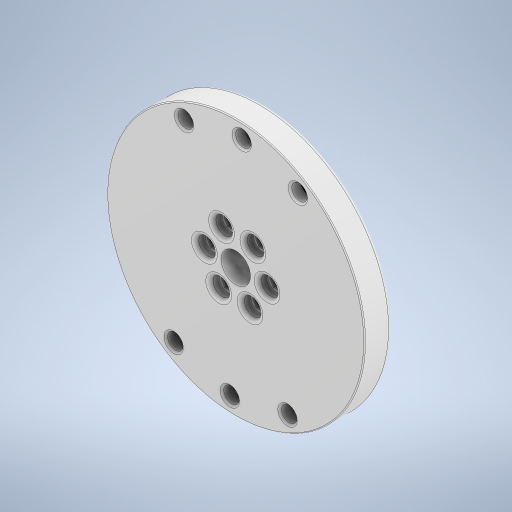
# Autodesk Inventor part: Góra
Saved by Autodesk Inventor 2023 (Build 270158000, 158)
## iProperties
Created: 2022-12-12
Part Number: Góra
Material: Stal, stopowa
Document SubType Name: Modeling
Designer: komputer
Density: 7.73 g/cm^3
Appearance: Gładki — biały
Author: komputer
Autodesk Inventor part; units mm, degrees
(part 1 of 2)
ref_plane "YZ Plane" through (0, 0, 0) normal (1, 0, 0) x (0, 1, 0)
ref_plane "XZ Plane" through (0, 0, 0) normal (0, 1, 0) x (-1, 0, 0)
sketch "Sketch1" plane through (0, 0, 0) normal (0, 0, 1) x (1, 0, 0)
  circle A0 centre (-9.064195, 40.309091) radius 2
  circle A1 centre (-10.61138, 10.787058) radius 2
  circle A2 centre (15.729043, 24.208174) radius 2
  circle A3 centre (6.433174, 9.893791) radius 2
  circle A4 centre (-18.360064, 25.994708) radius 2
  circle A5 centre (7.980358, 39.415824) radius 2
  circle A6 centre (-1.315511, 25.101441) radius 9
  circle A7 centre (-1.315511, 25.101441) radius 24.135889
  circle A8 centre (-1.315511, 25.101441) radius 25
  circle A9 centre (-9.064195, 40.309091) radius 3.5
  circle A10 centre (-10.61138, 10.787058) radius 3.5
  circle A11 centre (15.729043, 24.208174) radius 3.5
  circle A12 centre (6.433174, 9.893791) radius 3.5
  circle A13 centre (-18.360064, 25.994708) radius 3.5
  circle A14 centre (7.980358, 39.415824) radius 3.5
  arc A15 (-0.870133, 59.093921) -> (-1.760889, 59.093921) centre (-1.315511, 25.101441) ccw
  arc A16 (1.794733, 58.954262) -> (-0.870133, 59.093921) centre (-1.315511, 25.101441) ccw
  arc A17 (2.680609, 58.861152) -> (1.794733, 58.954262) centre (-1.315511, 25.101441) ccw
  arc A18 (5.316278, 58.443703) -> (2.680609, 58.861152) centre (-1.315511, 25.101441) ccw
  arc A19 (6.187569, 58.258505) -> (5.316278, 58.443703) centre (-1.315511, 25.101441) ccw
  arc A20 (8.765164, 57.56784) -> (6.187569, 58.258505) centre (-1.315511, 25.101441) ccw
  arc A21 (9.612323, 57.292581) -> (8.765164, 57.56784) centre (-1.315511, 25.101441) ccw
  arc A22 (12.103603, 56.336269) -> (9.612323, 57.292581) centre (-1.315511, 25.101441) ccw
  arc A23 (12.91735, 55.973965) -> (12.103603, 56.336269) centre (-1.315511, 25.101441) ccw
  arc A24 (15.295021, 54.762481) -> (12.91735, 55.973965) centre (-1.315511, 25.101441) ccw
  arc A25 (16.066438, 54.317103) -> (15.295021, 54.762481) centre (-1.315511, 25.101441) ccw
  arc A26 (18.304449, 52.863722) -> (16.066438, 54.317103) centre (-1.315511, 25.101441) ccw
  arc A27 (19.025086, 52.340149) -> (18.304449, 52.863722) centre (-1.315511, 25.101441) ccw
  arc A28 (21.098918, 50.660793) -> (19.025086, 52.340149) centre (-1.315511, 25.101441) ccw
  arc A29 (21.760878, 50.064761) -> (21.098918, 50.660793) centre (-1.315511, 25.101441) ccw
  arc A30 (23.647809, 48.17783) -> (21.760878, 50.064761) centre (-1.315511, 25.101441) ccw
  arc A31 (24.243841, 47.51587) -> (23.647809, 48.17783) centre (-1.315511, 25.101441) ccw
  arc A32 (25.923197, 45.442038) -> (24.243841, 47.51587) centre (-1.315511, 25.101441) ccw
  arc A33 (26.44677, 44.721401) -> (25.923197, 45.442038) centre (-1.315511, 25.101441) ccw
  arc A34 (27.900152, 42.48339) -> (26.44677, 44.721401) centre (-1.315511, 25.101441) ccw
  arc A35 (28.34553, 41.711972) -> (27.900152, 42.48339) centre (-1.315511, 25.101441) ccw
  arc A36 (29.557014, 39.334301) -> (28.34553, 41.711972) centre (-1.315511, 25.101441) ccw
  arc A37 (29.919317, 38.520555) -> (29.557014, 39.334301) centre (-1.315511, 25.101441) ccw
  arc A38 (30.87563, 36.029275) -> (29.919317, 38.520555) centre (-1.315511, 25.101441) ccw
  arc A39 (31.150888, 35.182115) -> (30.87563, 36.029275) centre (-1.315511, 25.101441) ccw
  arc A40 (31.841553, 32.604521) -> (31.150888, 35.182115) centre (-1.315511, 25.101441) ccw
  arc A41 (32.026751, 31.73323) -> (31.841553, 32.604521) centre (-1.315511, 25.101441) ccw
  arc A42 (32.4442, 29.097561) -> (32.026751, 31.73323) centre (-1.315511, 25.101441) ccw
  arc A43 (32.53731, 28.211685) -> (32.4442, 29.097561) centre (-1.315511, 25.101441) ccw
  arc A44 (32.676969, 25.546819) -> (32.53731, 28.211685) centre (-1.315511, 25.101441) ccw
  arc A45 (32.676969, 24.656063) -> (32.676969, 25.546819) centre (-1.315511, 25.101441) ccw
  arc A46 (32.53731, 21.991198) -> (32.676969, 24.656063) centre (-1.315511, 25.101441) ccw
  arc A47 (32.4442, 21.105321) -> (32.53731, 21.991198) centre (-1.315511, 25.101441) ccw
  arc A48 (32.026751, 18.469653) -> (32.4442, 21.105321) centre (-1.315511, 25.101441) ccw
  arc A49 (31.841553, 17.598362) -> (32.026751, 18.469653) centre (-1.315511, 25.101441) ccw
  arc A50 (31.150888, 15.020767) -> (31.841553, 17.598362) centre (-1.315511, 25.101441) ccw
  arc A51 (30.87563, 14.173607) -> (31.150888, 15.020767) centre (-1.315511, 25.101441) ccw
  arc A52 (29.919317, 11.682327) -> (30.87563, 14.173607) centre (-1.315511, 25.101441) ccw
  arc A53 (29.557014, 10.868581) -> (29.919317, 11.682327) centre (-1.315511, 25.101441) ccw
  arc A54 (28.34553, 8.49091) -> (29.557014, 10.868581) centre (-1.315511, 25.101441) ccw
  arc A55 (27.900152, 7.719492) -> (28.34553, 8.49091) centre (-1.315511, 25.101441) ccw
  arc A56 (26.44677, 5.481481) -> (27.900152, 7.719492) centre (-1.315511, 25.101441) ccw
  arc A57 (25.923197, 4.760844) -> (26.44677, 5.481481) centre (-1.315511, 25.101441) ccw
  arc A58 (24.243841, 2.687013) -> (25.923197, 4.760844) centre (-1.315511, 25.101441) ccw
  arc A59 (23.647809, 2.025052) -> (24.243841, 2.687013) centre (-1.315511, 25.101441) ccw
  arc A60 (21.760878, 0.138121) -> (23.647809, 2.025052) centre (-1.315511, 25.101441) ccw
  arc A61 (21.098918, -0.457911) -> (21.760878, 0.138121) centre (-1.315511, 25.101441) ccw
  arc A62 (19.025086, -2.137266) -> (21.098918, -0.457911) centre (-1.315511, 25.101441) ccw
  arc A63 (18.304449, -2.66084) -> (19.025086, -2.137266) centre (-1.315511, 25.101441) ccw
  arc A64 (16.066438, -4.114221) -> (18.304449, -2.66084) centre (-1.315511, 25.101441) ccw
  arc A65 (15.295021, -4.559599) -> (16.066438, -4.114221) centre (-1.315511, 25.101441) ccw
  arc A66 (12.91735, -5.771083) -> (15.295021, -4.559599) centre (-1.315511, 25.101441) ccw
  arc A67 (12.103603, -6.133386) -> (12.91735, -5.771083) centre (-1.315511, 25.101441) ccw
  arc A68 (9.612323, -7.089699) -> (12.103603, -6.133386) centre (-1.315511, 25.101441) ccw
  arc A69 (8.765164, -7.364958) -> (9.612323, -7.089699) centre (-1.315511, 25.101441) ccw
  arc A70 (6.187569, -8.055623) -> (8.765164, -7.364958) centre (-1.315511, 25.101441) ccw
  arc A71 (5.316278, -8.240821) -> (6.187569, -8.055623) centre (-1.315511, 25.101441) ccw
  arc A72 (2.680609, -8.65827) -> (5.316278, -8.240821) centre (-1.315511, 25.101441) ccw
  arc A73 (1.794733, -8.751379) -> (2.680609, -8.65827) centre (-1.315511, 25.101441) ccw
  arc A74 (-0.870133, -8.891039) -> (1.794733, -8.751379) centre (-1.315511, 25.101441) ccw
  arc A75 (-1.760889, -8.891039) -> (-0.870133, -8.891039) centre (-1.315511, 25.101441) ccw
  arc A76 (-4.425754, -8.751379) -> (-1.760889, -8.891039) centre (-1.315511, 25.101441) ccw
  arc A77 (-5.311631, -8.65827) -> (-4.425754, -8.751379) centre (-1.315511, 25.101441) ccw
  arc A78 (-7.947299, -8.240821) -> (-5.311631, -8.65827) centre (-1.315511, 25.101441) ccw
  arc A79 (-8.81859, -8.055623) -> (-7.947299, -8.240821) centre (-1.315511, 25.101441) ccw
  arc A80 (-11.396185, -7.364958) -> (-8.81859, -8.055623) centre (-1.315511, 25.101441) ccw
  arc A81 (-12.243345, -7.089699) -> (-11.396185, -7.364958) centre (-1.315511, 25.101441) ccw
  arc A82 (-14.734625, -6.133386) -> (-12.243345, -7.089699) centre (-1.315511, 25.101441) ccw
  arc A83 (-15.548371, -5.771083) -> (-14.734625, -6.133386) centre (-1.315511, 25.101441) ccw
  arc A84 (-17.926042, -4.559599) -> (-15.548371, -5.771083) centre (-1.315511, 25.101441) ccw
  arc A85 (-18.69746, -4.114221) -> (-17.926042, -4.559599) centre (-1.315511, 25.101441) ccw
  arc A86 (-20.935471, -2.66084) -> (-18.69746, -4.114221) centre (-1.315511, 25.101441) ccw
  arc A87 (-21.656108, -2.137266) -> (-20.935471, -2.66084) centre (-1.315511, 25.101441) ccw
  arc A88 (-23.729939, -0.457911) -> (-21.656108, -2.137266) centre (-1.315511, 25.101441) ccw
  arc A89 (-24.3919, 0.138121) -> (-23.729939, -0.457911) centre (-1.315511, 25.101441) ccw
  arc A90 (-26.27883, 2.025052) -> (-24.3919, 0.138121) centre (-1.315511, 25.101441) ccw
  arc A91 (-26.874863, 2.687013) -> (-26.27883, 2.025052) centre (-1.315511, 25.101441) ccw
  arc A92 (-28.554218, 4.760844) -> (-26.874863, 2.687013) centre (-1.315511, 25.101441) ccw
  arc A93 (-29.077792, 5.481481) -> (-28.554218, 4.760844) centre (-1.315511, 25.101441) ccw
  arc A94 (-30.531173, 7.719492) -> (-29.077792, 5.481481) centre (-1.315511, 25.101441) ccw
  arc A95 (-30.976551, 8.49091) -> (-30.531173, 7.719492) centre (-1.315511, 25.101441) ccw
  arc A96 (-32.188035, 10.868581) -> (-30.976551, 8.49091) centre (-1.315511, 25.101441) ccw
  arc A97 (-32.550338, 11.682327) -> (-32.188035, 10.868581) centre (-1.315511, 25.101441) ccw
  arc A98 (-33.506651, 14.173607) -> (-32.550338, 11.682327) centre (-1.315511, 25.101441) ccw
  arc A99 (-33.78191, 15.020767) -> (-33.506651, 14.173607) centre (-1.315511, 25.101441) ccw
  arc A100 (-34.472574, 17.598362) -> (-33.78191, 15.020767) centre (-1.315511, 25.101441) ccw
  arc A101 (-34.657773, 18.469653) -> (-34.472574, 17.598362) centre (-1.315511, 25.101441) ccw
  arc A102 (-35.075222, 21.105321) -> (-34.657773, 18.469653) centre (-1.315511, 25.101441) ccw
  arc A103 (-35.168331, 21.991198) -> (-35.075222, 21.105321) centre (-1.315511, 25.101441) ccw
  arc A104 (-35.307991, 24.656063) -> (-35.168331, 21.991198) centre (-1.315511, 25.101441) ccw
  arc A105 (-35.307991, 25.546819) -> (-35.307991, 24.656063) centre (-1.315511, 25.101441) ccw
  arc A106 (-35.168331, 28.211685) -> (-35.307991, 25.546819) centre (-1.315511, 25.101441) ccw
  arc A107 (-35.075222, 29.097561) -> (-35.168331, 28.211685) centre (-1.315511, 25.101441) ccw
  arc A108 (-34.657773, 31.73323) -> (-35.075222, 29.097561) centre (-1.315511, 25.101441) ccw
  arc A109 (-34.472574, 32.604521) -> (-34.657773, 31.73323) centre (-1.315511, 25.101441) ccw
  arc A110 (-33.78191, 35.182115) -> (-34.472574, 32.604521) centre (-1.315511, 25.101441) ccw
  arc A111 (-33.506651, 36.029275) -> (-33.78191, 35.182115) centre (-1.315511, 25.101441) ccw
  arc A112 (-32.550338, 38.520555) -> (-33.506651, 36.029275) centre (-1.315511, 25.101441) ccw
  arc A113 (-32.188035, 39.334301) -> (-32.550338, 38.520555) centre (-1.315511, 25.101441) ccw
  arc A114 (-30.976551, 41.711972) -> (-32.188035, 39.334301) centre (-1.315511, 25.101441) ccw
  arc A115 (-30.531173, 42.48339) -> (-30.976551, 41.711972) centre (-1.315511, 25.101441) ccw
  arc A116 (-29.077792, 44.721401) -> (-30.531173, 42.48339) centre (-1.315511, 25.101441) ccw
  arc A117 (-28.554218, 45.442038) -> (-29.077792, 44.721401) centre (-1.315511, 25.101441) ccw
  arc A118 (-26.874863, 47.51587) -> (-28.554218, 45.442038) centre (-1.315511, 25.101441) ccw
  arc A119 (-26.27883, 48.17783) -> (-26.874863, 47.51587) centre (-1.315511, 25.101441) ccw
  arc A120 (-24.3919, 50.064761) -> (-26.27883, 48.17783) centre (-1.315511, 25.101441) ccw
  arc A121 (-23.729939, 50.660793) -> (-24.3919, 50.064761) centre (-1.315511, 25.101441) ccw
  arc A122 (-21.656108, 52.340149) -> (-23.729939, 50.660793) centre (-1.315511, 25.101441) ccw
  arc A123 (-20.935471, 52.863722) -> (-21.656108, 52.340149) centre (-1.315511, 25.101441) ccw
  arc A124 (-18.69746, 54.317103) -> (-20.935471, 52.863722) centre (-1.315511, 25.101441) ccw
  arc A125 (-17.926042, 54.762481) -> (-18.69746, 54.317103) centre (-1.315511, 25.101441) ccw
  arc A126 (-15.548371, 55.973965) -> (-17.926042, 54.762481) centre (-1.315511, 25.101441) ccw
  arc A127 (-14.734625, 56.336269) -> (-15.548371, 55.973965) centre (-1.315511, 25.101441) ccw
  arc A128 (-12.243345, 57.292581) -> (-14.734625, 56.336269) centre (-1.315511, 25.101441) ccw
  arc A129 (-11.396185, 57.56784) -> (-12.243345, 57.292581) centre (-1.315511, 25.101441) ccw
  arc A130 (-8.81859, 58.258505) -> (-11.396185, 57.56784) centre (-1.315511, 25.101441) ccw
  arc A131 (-7.947299, 58.443703) -> (-8.81859, 58.258505) centre (-1.315511, 25.101441) ccw
  arc A132 (-5.311631, 58.861152) -> (-7.947299, 58.443703) centre (-1.315511, 25.101441) ccw
  arc A133 (-4.425754, 58.954262) -> (-5.311631, 58.861152) centre (-1.315511, 25.101441) ccw
  arc A134 (-1.760889, 59.093921) -> (-4.425754, 58.954262) centre (-1.315511, 25.101441) ccw
  circle A135 centre (-1.315511, 25.101441) radius 9
  circle A136 centre (-1.315511, 25.101441) radius 8
  point P0 (0, 0)
extrude "Extrusion1" add sketch "Sketch1" along normal blind 37 contours A6 | A7 | A9 | A10 | A11 | A12 | A13 | A14
sketch "Sketch2" plane through (-1.315511, 25.101441, 37) normal (0, 0, 1) x (1, 0, 0)
  circle A0 centre (0, 0) radius 43.680391
  circle A1 centre (0, 0) radius 8
  circle A2 centre (0, 0) radius 50
  circle A3 centre (0, 0) radius 24.135889
  circle A4 centre (9.295869, 14.314383) radius 2
  circle A5 centre (-17.044553, 0.893267) radius 2
  circle A6 centre (7.748685, -15.20765) radius 2
  circle A7 centre (17.044553, -0.893267) radius 2
  circle A8 centre (-9.295869, -14.314383) radius 2
  circle A9 centre (-7.748685, 15.20765) radius 2
  circle A10 centre (0, 0) radius 8
  point P0 (1.315511, -25.101441)
  dimension "d2" = 100
  constraints: 1 centre point, 1 coincident
  measures "d2" diameter of A2
extrude "Extrusion2" add sketch "Sketch2" against normal blind 10 contours A0 | A2
sketch "Sketch3" plane through (-1.315511, 25.101441, 37) normal (0, 0, 1) x (1, 0, 0)
  circle A0 centre (0, 0) radius 55
  circle A1 centre (0, 0) radius 50
  circle A2 centre (9.295869, 14.314383) radius 2
  circle A3 centre (-17.044553, 0.893267) radius 2
  circle A4 centre (7.748685, -15.20765) radius 2
  circle A5 centre (17.044553, -0.893267) radius 2
  circle A6 centre (-9.295869, -14.314383) radius 2
  circle A7 centre (-7.748685, 15.20765) radius 2
  circle A8 centre (0, 0) radius 8
  point P0 (1.315511, -25.101441)
  constraints: 1 centre point, 2 other
ref_plane "Work Plane1" through (-65.256929, -38.839977, 26) normal (0, 0, 1) x (0.9839108, 0.1786605, 0)
extrude "Extrusion3" add sketch "Sketch3" against normal blind 10 contours A0
sketch "Sketch4" plane through (-1.315511, 25.101441, 37) normal (0, 0, 1) x (1, 0, 0)
  circle A0 centre (0, 0) radius 55
  circle A1 centre (9.295869, 14.314383) radius 2
  circle A2 centre (-17.044553, 0.893267) radius 2
  circle A3 centre (7.748685, -15.20765) radius 2
  circle A4 centre (17.044553, -0.893267) radius 2
  circle A5 centre (-9.295869, -14.314383) radius 2
  circle A6 centre (-7.748685, 15.20765) radius 2
  circle A7 centre (0, 0) radius 8
  line L0 (-9.295869, -14.314383) -> (-9.295869, -10.814383)
  line L1 (-9.295869, -10.814383) -> (-9.295869, -17.414383)
  line L2 (-11.085655, -17.414383) -> (-12.87544, -14.314383)
  line L3 (-12.87544, -14.314383) -> (-11.085655, -11.214383)
  line L4 (-11.085655, -11.214383) -> (-7.506083, -11.214383)
  line L5 (-7.506083, -11.214383) -> (-5.716297, -14.314383)
  line L6 (-5.716297, -14.314383) -> (-7.506083, -17.414383)
  line L7 (-7.506083, -17.414383) -> (-11.085655, -17.414383)
  line L8 (9.53847, -12.10765) -> (11.328256, -15.20765)
  line L9 (9.53847, -18.30765) -> (5.958899, -18.30765)
  line L10 (5.958899, -18.30765) -> (4.169113, -15.20765)
  line L11 (11.328256, -15.20765) -> (9.53847, -18.30765)
  line L12 (4.169113, -15.20765) -> (5.958899, -12.10765)
  line L13 (5.958899, -12.10765) -> (9.53847, -12.10765)
  line L14 (15.254768, 2.206733) -> (18.834339, 2.206733)
  line L15 (20.624125, -0.893267) -> (18.834339, -3.993267)
  line L16 (18.834339, -3.993267) -> (15.254768, -3.993267)
  line L17 (18.834339, 2.206733) -> (20.624125, -0.893267)
  line L18 (15.254768, -3.993267) -> (13.464982, -0.893267)
  line L19 (13.464982, -0.893267) -> (15.254768, 2.206733)
  line L20 (5.716297, 14.314383) -> (7.506083, 17.414383)
  line L21 (11.085655, 17.414383) -> (12.87544, 14.314383)
  line L22 (12.87544, 14.314383) -> (11.085655, 11.214383)
  line L23 (7.506083, 17.414383) -> (11.085655, 17.414383)
  line L24 (11.085655, 11.214383) -> (7.506083, 11.214383)
  line L25 (7.506083, 11.214383) -> (5.716297, 14.314383)
  line L26 (-9.53847, 12.10765) -> (-11.328256, 15.20765)
  line L27 (-9.53847, 18.30765) -> (-5.958899, 18.30765)
  line L28 (-5.958899, 18.30765) -> (-4.169113, 15.20765)
  line L29 (-11.328256, 15.20765) -> (-9.53847, 18.30765)
  line L30 (-4.169113, 15.20765) -> (-5.958899, 12.10765)
  line L31 (-5.958899, 12.10765) -> (-9.53847, 12.10765)
  line L32 (-15.254768, -2.206733) -> (-18.834339, -2.206733)
  line L33 (-20.624125, 0.893267) -> (-18.834339, 3.993267)
  line L34 (-18.834339, 3.993267) -> (-15.254768, 3.993267)
  line L35 (-18.834339, -2.206733) -> (-20.624125, 0.893267)
  line L36 (-15.254768, 3.993267) -> (-13.464982, 0.893267)
  line L37 (-13.464982, 0.893267) -> (-15.254768, -2.206733)
  point P0 (1.315511, -25.101441)
  point P1 (10.433363, -16.75765)
  point P2 (7.748685, -15.20765)
  point P3 (4.717596, -13.45765)
  point P4 (19.729232, 0.656733)
  point P5 (17.044553, -0.893267)
  point P6 (14.013465, -2.643267)
  point P7 (9.295869, 17.414383)
  point P8 (9.295869, 14.314383)
  point P9 (9.295869, 10.814383)
  point P10 (-10.433363, 16.75765)
  point P11 (-7.748685, 15.20765)
  point P12 (-4.717596, 13.45765)
  point P13 (-19.729232, -0.656733)
  point P14 (-17.044553, 0.893267)
  point P15 (-14.013465, 2.643267)
  dimension "d7" = 3.5
  dimension "d8" = 6.6
  dimension "d11" = 360
  constraints: 76 end point, 2 coincident, 1 midpoint, 1 point on line, 1 vertical, 104 other
  measures "d7" distance of L0.start L0.end
  measures "d8" distance of L0.end L1.end
extrude "Extrusion4" cut sketch "Sketch4" against normal blind 5.4 contours A1 | A2 | A3 | A4 | A5 L1 L0 | A5 L0 L4 L5 L6 L7 L1 | L0 L1 A5 | A5 L1 L7 L2 L3 L4 L0 | A6 | L8 L11 L9 L10 L12 L13 | L14 L17 L15 L16 L18 L19 | L20 L23 L21 L22 L24 L25 | L26 L29 L27 L28 L30 L31 | L32 L35 L33 L34 L36 L37
sketch "Sketch14" plane through (-1.315511, 25.101441, 37) normal (0, 0, 1) x (1, 0, 0)
  circle A0 centre (0, 0) radius 55
  line L0 (-7.506083, -11.214383) -> (-5.716297, -14.314383)
  line L1 (-5.716297, -14.314383) -> (-7.506083, -17.414383)
  line L2 (-7.506083, -17.414383) -> (-11.085655, -17.414383)
  line L3 (-11.085655, -17.414383) -> (-12.87544, -14.314383)
  line L4 (-12.87544, -14.314383) -> (-11.085655, -11.214383)
  line L5 (-11.085655, -11.214383) -> (-7.506083, -11.214383)
  line L6 (18.834339, -3.993267) -> (15.254768, -3.993267)
  line L7 (15.254768, -3.993267) -> (13.464982, -0.893267)
  line L8 (13.464982, -0.893267) -> (15.254768, 2.206733)
  line L9 (15.254768, 2.206733) -> (18.834339, 2.206733)
  line L10 (18.834339, 2.206733) -> (20.624125, -0.893267)
  line L11 (20.624125, -0.893267) -> (18.834339, -3.993267)
  line L12 (12.87544, 14.314383) -> (11.085655, 11.214383)
  line L13 (11.085655, 11.214383) -> (7.506083, 11.214383)
  line L14 (7.506083, 11.214383) -> (5.716297, 14.314383)
  line L15 (5.716297, 14.314383) -> (7.506083, 17.414383)
  line L16 (7.506083, 17.414383) -> (11.085655, 17.414383)
  line L17 (11.085655, 17.414383) -> (12.87544, 14.314383)
  line L18 (-18.834339, 3.993267) -> (-15.254768, 3.993267)
  line L19 (-15.254768, 3.993267) -> (-13.464982, 0.893267)
  line L20 (-13.464982, 0.893267) -> (-15.254768, -2.206733)
  line L21 (-15.254768, -2.206733) -> (-18.834339, -2.206733)
  line L22 (-18.834339, -2.206733) -> (-20.624125, 0.893267)
  line L23 (-20.624125, 0.893267) -> (-18.834339, 3.993267)
  line L24 (5.958899, -18.30765) -> (4.169113, -15.20765)
  line L25 (4.169113, -15.20765) -> (5.958899, -12.10765)
  line L26 (5.958899, -12.10765) -> (9.53847, -12.10765)
  line L27 (9.53847, -12.10765) -> (11.328256, -15.20765)
  line L28 (11.328256, -15.20765) -> (9.53847, -18.30765)
  line L29 (9.53847, -18.30765) -> (5.958899, -18.30765)
  line L30 (-5.958899, 18.30765) -> (-4.169113, 15.20765)
  line L31 (-4.169113, 15.20765) -> (-5.958899, 12.10765)
  line L32 (-5.958899, 12.10765) -> (-9.53847, 12.10765)
  line L33 (-9.53847, 12.10765) -> (-11.328256, 15.20765)
  line L34 (-11.328256, 15.20765) -> (-9.53847, 18.30765)
  line L35 (-9.53847, 18.30765) -> (-5.958899, 18.30765)
  circle A1 centre (-9.295869, -14.314383) radius 2
  circle A2 centre (7.748685, -15.20765) radius 2
  circle A3 centre (9.295869, 14.314383) radius 2
  circle A4 centre (-7.748685, 15.20765) radius 2
  circle A5 centre (7.748685, -15.20765) radius 2
  line L36 (-9.295869, -14.314383) -> (7.748685, -15.20765)
  line L37 (-7.748685, 15.20765) -> (9.295869, 14.314383)
  line L38 (0, 0) -> (-0.773592, -14.761016)
  line L39 (0, 0) -> (0.773592, 14.761016)
  line L40 (0, 0) -> (2.355118, 44.938329)
  circle A6 centre (0, 0) radius 8
  line L41 (0, 0) -> (-2.355118, -44.938329)
  line L42 (-2.355118, -44.938329) -> (-54.509523, -42.205033)
  line L43 (-54.509523, -42.205033) -> (48.627627, -47.610222)
  line L44 (2.355118, 44.938329) -> (-54.509523, 47.918479)
  line L45 (2.355118, 44.938329) -> (72.939254, 41.239171)
  line L46 (2.355118, 44.938329) -> (3.506509, 66.908179)
  line L47 (0, 0) -> (-7.748685, 15.20765)
  line L48 (-7.748685, 15.20765) -> (-23.590038, 46.298057)
  line L49 (-23.590038, 46.298057) -> (-32.669848, 64.118188)
  circle A7 centre (0, 0) radius 71.961524
  circle A8 centre (-28.129943, 55.208122) radius 4
  circle A9 centre (-51.965307, 33.746665) radius 4
  circle A10 centre (-61.876608, 3.242816) radius 4
  circle A11 centre (-55.208122, -28.129943) radius 4
  circle A12 centre (-33.746665, -51.965307) radius 4
  circle A13 centre (-3.242816, -61.876608) radius 4
  circle A14 centre (28.129943, -55.208122) radius 4
  circle A15 centre (51.965307, -33.746665) radius 4
  circle A16 centre (61.876608, -3.242816) radius 4
  circle A17 centre (55.208122, 28.129943) radius 4
  circle A18 centre (33.746665, 51.965307) radius 4
  circle A19 centre (3.242816, 61.876608) radius 4
  line L50 (-2.355118, -44.938329) -> (-68.6558, -41.463658)
  line L51 (-68.6558, -41.463658) -> (71.961524, -48.833099)
  point P0 (1.315511, -25.101441)
  dimension "d60" = 45
  dimension "d61" = 45
  dimension "d62" = 22
  dimension "d63" = 20
  dimension "d65" = 8
  dimension "d69" = 360
  constraints: 32 end point, 12 centre point, 3 collinear, 3 midpoint, 3 perpendicular, 3 point on line, 2 coincident, 28 other
  measures "d60" distance of L38.start L40.end
  measures "d61" distance of L41.start L41.end
  measures "d62" distance of L40.end L46.end
  measures "d63" distance of L48.end L49.end
  measures "d65" diameter of A8
extrude "Extrusion16" add sketch "Sketch14" against normal up to surface (10 mm away) contours A0 L45 A7 L51 L43 | A0 L49 A8 A7 L45 | L43 L51 A7 L50 L42 A0 | L42 L50 A7 L44 A0 | A0 L44 A7 L49 A8 | A9 | A10 | A11 | A15 | A16 | A17
sketch "Sketch15" plane through (-1.315511, 25.101441, 37) normal (0, 0, 1) x (1, 0, 0)
  circle A0 centre (-28.129943, 55.208122) radius 4
  circle A1 centre (33.746665, 51.965307) radius 4
  circle A2 centre (-33.746665, -51.965307) radius 4
  circle A3 centre (-3.242816, -61.876608) radius 4
  circle A4 centre (28.129943, -55.208122) radius 4
  circle A5 centre (3.242816, 61.876608) radius 4
  circle A6 centre (0, 0) radius 71.961524
  line L0 (-7.506083, -11.214383) -> (-5.716297, -14.314383)
  line L1 (-5.716297, -14.314383) -> (-7.506083, -17.414383)
  line L2 (-7.506083, -17.414383) -> (-11.085655, -17.414383)
  line L3 (-11.085655, -17.414383) -> (-12.87544, -14.314383)
  line L4 (-12.87544, -14.314383) -> (-11.085655, -11.214383)
  line L5 (-11.085655, -11.214383) -> (-7.506083, -11.214383)
  line L6 (18.834339, -3.993267) -> (15.254768, -3.993267)
  line L7 (15.254768, -3.993267) -> (13.464982, -0.893267)
  line L8 (13.464982, -0.893267) -> (15.254768, 2.206733)
  line L9 (15.254768, 2.206733) -> (18.834339, 2.206733)
  line L10 (18.834339, 2.206733) -> (20.624125, -0.893267)
  line L11 (20.624125, -0.893267) -> (18.834339, -3.993267)
  line L12 (12.87544, 14.314383) -> (11.085655, 11.214383)
  line L13 (11.085655, 11.214383) -> (7.506083, 11.214383)
  line L14 (7.506083, 11.214383) -> (5.716297, 14.314383)
  line L15 (5.716297, 14.314383) -> (7.506083, 17.414383)
  line L16 (7.506083, 17.414383) -> (11.085655, 17.414383)
  line L17 (11.085655, 17.414383) -> (12.87544, 14.314383)
  line L18 (-18.834339, 3.993267) -> (-15.254768, 3.993267)
  line L19 (-15.254768, 3.993267) -> (-13.464982, 0.893267)
  line L20 (-13.464982, 0.893267) -> (-15.254768, -2.206733)
  line L21 (-15.254768, -2.206733) -> (-18.834339, -2.206733)
  line L22 (-18.834339, -2.206733) -> (-20.624125, 0.893267)
  line L23 (-20.624125, 0.893267) -> (-18.834339, 3.993267)
  line L24 (5.958899, -18.30765) -> (4.169113, -15.20765)
  line L25 (4.169113, -15.20765) -> (5.958899, -12.10765)
  line L26 (5.958899, -12.10765) -> (9.53847, -12.10765)
  line L27 (9.53847, -12.10765) -> (11.328256, -15.20765)
  line L28 (11.328256, -15.20765) -> (9.53847, -18.30765)
  line L29 (9.53847, -18.30765) -> (5.958899, -18.30765)
  line L30 (-5.958899, 18.30765) -> (-4.169113, 15.20765)
  line L31 (-4.169113, 15.20765) -> (-5.958899, 12.10765)
  line L32 (-5.958899, 12.10765) -> (-9.53847, 12.10765)
  line L33 (-9.53847, 12.10765) -> (-11.328256, 15.20765)
  line L34 (-11.328256, 15.20765) -> (-9.53847, 18.30765)
  line L35 (-9.53847, 18.30765) -> (-5.958899, 18.30765)
  circle A7 centre (0, 0) radius 70
  point P0 (1.315511, -25.101441)
  dimension "d73" = 140
  constraints: 1 centre point
  measures "d73" diameter of A7
extrude "Extrusion17" cut sketch "Sketch15" against normal through all contours A6
sketch "Sketch16" plane through (-1.315511, 25.101441, 27) normal (0, 0, -1) x (-1, 0, 0)
  circle A0 centre (0, 0) radius 70
  circle A1 centre (-3.242816, 61.876608) radius 4
  circle A2 centre (-28.129943, -55.208122) radius 4
  circle A3 centre (3.242816, -61.876608) radius 4
  circle A4 centre (33.746665, -51.965307) radius 4
  circle A5 centre (-33.746665, 51.965307) radius 4
  circle A6 centre (28.129943, 55.208122) radius 4
  circle A7 centre (0, 0) radius 24.135889
  circle A8 centre (-28.129943, -55.208122) radius 4
  circle A9 centre (28.129943, 55.208122) radius 4
  line L0 (-28.129943, -55.208122) -> (28.129943, 55.208122)
  line L1 (-28.129943, -55.208122) -> (-25.315202, -49.683882)
  line L2 (-22.125781, -51.308973) -> (-21.7511, -58.458305)
  line L3 (-21.7511, -58.458305) -> (-27.755263, -62.357454)
  line L4 (-27.755263, -62.357454) -> (-34.134106, -59.107271)
  line L5 (-34.134106, -59.107271) -> (-34.508787, -51.957939)
  line L6 (-34.508787, -51.957939) -> (-28.504624, -48.05879)
  line L7 (-28.504624, -48.05879) -> (-22.125781, -51.308973)
  line L8 (-0.656333, -55.872445) -> (6.492999, -55.497765)
  line L9 (-3.906516, -62.251289) -> (-0.656333, -55.872445)
  line L10 (-0.007367, -68.255452) -> (-3.906516, -62.251289)
  line L11 (7.141965, -67.880771) -> (-0.007367, -68.255452)
  line L12 (10.392148, -61.501927) -> (7.141965, -67.880771)
  line L13 (6.492999, -55.497765) -> (10.392148, -61.501927)
  line L14 (27.367821, -48.715124) -> (33.371984, -44.815975)
  line L15 (27.742502, -55.864456) -> (27.367821, -48.715124)
  line L16 (34.121345, -59.114639) -> (27.742502, -55.864456)
  line L17 (40.125508, -55.21549) -> (34.121345, -59.114639)
  line L18 (39.750828, -48.066158) -> (40.125508, -55.21549)
  line L19 (33.371984, -44.815975) -> (39.750828, -48.066158)
  line L20 (48.05879, -28.504624) -> (51.308973, -22.125781)
  line L21 (51.957939, -34.508787) -> (48.05879, -28.504624)
  line L22 (59.107271, -34.134106) -> (51.957939, -34.508787)
  line L23 (62.357454, -27.755263) -> (59.107271, -34.134106)
  line L24 (58.458305, -21.7511) -> (62.357454, -27.755263)
  line L25 (51.308973, -22.125781) -> (58.458305, -21.7511)
  line L26 (55.872445, -0.656333) -> (55.497765, 6.492999)
  line L27 (62.251289, -3.906516) -> (55.872445, -0.656333)
  line L28 (68.255452, -0.007367) -> (62.251289, -3.906516)
  line L29 (67.880771, 7.141965) -> (68.255452, -0.007367)
  line L30 (61.501927, 10.392148) -> (67.880771, 7.141965)
  line L31 (55.497765, 6.492999) -> (61.501927, 10.392148)
  line L32 (48.715124, 27.367821) -> (44.815975, 33.371984)
  line L33 (55.864456, 27.742502) -> (48.715124, 27.367821)
  line L34 (59.114639, 34.121345) -> (55.864456, 27.742502)
  line L35 (55.21549, 40.125508) -> (59.114639, 34.121345)
  line L36 (48.066158, 39.750828) -> (55.21549, 40.125508)
  line L37 (44.815975, 33.371984) -> (48.066158, 39.750828)
  line L38 (28.504624, 48.05879) -> (22.125781, 51.308973)
  line L39 (34.508787, 51.957939) -> (28.504624, 48.05879)
  line L40 (34.134106, 59.107271) -> (34.508787, 51.957939)
  line L41 (27.755263, 62.357454) -> (34.134106, 59.107271)
  line L42 (21.7511, 58.458305) -> (27.755263, 62.357454)
  line L43 (22.125781, 51.308973) -> (21.7511, 58.458305)
  line L44 (0.656333, 55.872445) -> (-6.492999, 55.497765)
  line L45 (3.906516, 62.251289) -> (0.656333, 55.872445)
  line L46 (0.007367, 68.255452) -> (3.906516, 62.251289)
  line L47 (-7.141965, 67.880771) -> (0.007367, 68.255452)
  line L48 (-10.392148, 61.501927) -> (-7.141965, 67.880771)
  line L49 (-6.492999, 55.497765) -> (-10.392148, 61.501927)
  line L50 (-27.367821, 48.715124) -> (-33.371984, 44.815975)
  line L51 (-27.742502, 55.864456) -> (-27.367821, 48.715124)
  line L52 (-34.121345, 59.114639) -> (-27.742502, 55.864456)
  line L53 (-40.125508, 55.21549) -> (-34.121345, 59.114639)
  line L54 (-39.750828, 48.066158) -> (-40.125508, 55.21549)
  line L55 (-33.371984, 44.815975) -> (-39.750828, 48.066158)
  line L56 (-48.05879, 28.504624) -> (-51.308973, 22.125781)
  line L57 (-51.957939, 34.508787) -> (-48.05879, 28.504624)
  line L58 (-59.107271, 34.134106) -> (-51.957939, 34.508787)
  line L59 (-62.357454, 27.755263) -> (-59.107271, 34.134106)
  line L60 (-58.458305, 21.7511) -> (-62.357454, 27.755263)
  line L61 (-51.308973, 22.125781) -> (-58.458305, 21.7511)
  line L62 (-55.872445, 0.656333) -> (-55.497765, -6.492999)
  line L63 (-62.251289, 3.906516) -> (-55.872445, 0.656333)
  line L64 (-68.255452, 0.007367) -> (-62.251289, 3.906516)
  line L65 (-67.880771, -7.141965) -> (-68.255452, 0.007367)
  line L66 (-61.501927, -10.392148) -> (-67.880771, -7.141965)
  line L67 (-55.497765, -6.492999) -> (-61.501927, -10.392148)
  line L68 (-48.715124, -27.367821) -> (-44.815975, -33.371984)
  line L69 (-55.864456, -27.742502) -> (-48.715124, -27.367821)
  line L70 (-59.114639, -34.121345) -> (-55.864456, -27.742502)
  line L71 (-55.21549, -40.125508) -> (-59.114639, -34.121345)
  line L72 (-48.066158, -39.750828) -> (-55.21549, -40.125508)
  line L73 (-44.815975, -33.371984) -> (-48.066158, -39.750828)
  point P0 (-1.315511, -25.101441)
  point P1 (2.918333, -55.685105)
  point P2 (30.369903, -46.765549)
  point P3 (49.683882, -25.315202)
  point P4 (55.685105, 2.918333)
  point P5 (46.765549, 30.369903)
  point P6 (25.315202, 49.683882)
  point P7 (-2.918333, 55.685105)
  point P8 (-30.369903, 46.765549)
  point P9 (-49.683882, 25.315202)
  point P10 (-55.685105, -2.918333)
  point P11 (-46.765549, -30.369903)
  dimension "d76" = 6.2
  dimension "d79" = 360
  constraints: 148 end point, 1 coincident, 1 midpoint, 1 point on line, 170 other
  measures "d76" distance of L0.start L1.end
extrude "Extrusion18" cut sketch "Sketch16" against normal blind 9 contours A1 | A2 | A3 | A4 | A5 | A6 | L2 L3 L4 L5 L6 L7 | L8 L13 L12 L11 L10 L9 | L14 L19 L18 L17 L16 L15 | L38 L43 L42 L41 L40 L39 | L44 L49 L48 L47 L46 L45 | L50 L55 L54 L53 L52 L51
sketch "Sketch17" plane through (-1.315511, 25.101441, 37) normal (0, 0, 1) x (1, 0, 0)
  circle A0 centre (0, 0) radius 70
  circle A1 centre (-28.129943, 55.208122) radius 4
  circle A2 centre (33.746665, 51.965307) radius 4
  circle A3 centre (-33.746665, -51.965307) radius 4
  circle A4 centre (-3.242816, -61.876608) radius 4
  circle A5 centre (28.129943, -55.208122) radius 4
  circle A6 centre (3.242816, 61.876608) radius 4
  line L0 (-5.958899, 18.30765) -> (-4.169113, 15.20765)
  line L1 (-4.169113, 15.20765) -> (-5.958899, 12.10765)
  line L2 (-5.958899, 12.10765) -> (-9.53847, 12.10765)
  line L3 (-9.53847, 12.10765) -> (-11.328256, 15.20765)
  line L4 (-11.328256, 15.20765) -> (-9.53847, 18.30765)
  line L5 (-9.53847, 18.30765) -> (-5.958899, 18.30765)
  line L6 (5.958899, -18.30765) -> (4.169113, -15.20765)
  line L7 (4.169113, -15.20765) -> (5.958899, -12.10765)
  line L8 (5.958899, -12.10765) -> (9.53847, -12.10765)
  line L9 (9.53847, -12.10765) -> (11.328256, -15.20765)
  line L10 (11.328256, -15.20765) -> (9.53847, -18.30765)
  line L11 (9.53847, -18.30765) -> (5.958899, -18.30765)
  line L12 (-18.834339, 3.993267) -> (-15.254768, 3.993267)
  line L13 (-15.254768, 3.993267) -> (-13.464982, 0.893267)
  line L14 (-13.464982, 0.893267) -> (-15.254768, -2.206733)
  line L15 (-15.254768, -2.206733) -> (-18.834339, -2.206733)
  line L16 (-18.834339, -2.206733) -> (-20.624125, 0.893267)
  line L17 (-20.624125, 0.893267) -> (-18.834339, 3.993267)
  line L18 (12.87544, 14.314383) -> (11.085655, 11.214383)
  line L19 (11.085655, 11.214383) -> (7.506083, 11.214383)
  line L20 (7.506083, 11.214383) -> (5.716297, 14.314383)
  line L21 (5.716297, 14.314383) -> (7.506083, 17.414383)
  line L22 (7.506083, 17.414383) -> (11.085655, 17.414383)
  line L23 (11.085655, 17.414383) -> (12.87544, 14.314383)
  line L24 (18.834339, -3.993267) -> (15.254768, -3.993267)
  line L25 (15.254768, -3.993267) -> (13.464982, -0.893267)
  line L26 (13.464982, -0.893267) -> (15.254768, 2.206733)
  line L27 (15.254768, 2.206733) -> (18.834339, 2.206733)
  line L28 (18.834339, 2.206733) -> (20.624125, -0.893267)
  line L29 (20.624125, -0.893267) -> (18.834339, -3.993267)
  line L30 (-7.506083, -11.214383) -> (-5.716297, -14.314383)
  line L31 (-5.716297, -14.314383) -> (-7.506083, -17.414383)
  line L32 (-7.506083, -17.414383) -> (-11.085655, -17.414383)
  line L33 (-11.085655, -17.414383) -> (-12.87544, -14.314383)
  line L34 (-12.87544, -14.314383) -> (-11.085655, -11.214383)
  line L35 (-11.085655, -11.214383) -> (-7.506083, -11.214383)
  circle A7 centre (0, 0) radius 8
  point P0 (1.315511, -25.101441)
extrude "Extrusion19" add sketch "Sketch17" along normal blind 5
sketch "Sketch18" plane through (-1.315511, 25.101441, 0) normal (0, 0, -1) x (-1, 0, 0)
  circle A0 centre (0, 0) radius 24.135889
  circle A1 centre (-9.295869, 14.314383) radius 2
  circle A2 centre (17.044553, 0.893267) radius 2
  circle A3 centre (-7.748685, -15.20765) radius 2
  circle A4 centre (-17.044553, -0.893267) radius 2
  circle A5 centre (9.295869, -14.314383) radius 2
  circle A6 centre (7.748685, 15.20765) radius 2
  circle A7 centre (0, 0) radius 8
  point P0 (-1.315511, -25.101441)
extrude "Extrusion20" cut sketch "Sketch18" against normal blind 10
sketch "Sketch19" plane through (-1.315511, 25.101441, 10) normal (0, 0, -1) x (-1, 0, 0)
  circle A0 centre (0, 0) radius 24.135889
  circle A1 centre (0, 0) radius 8
  circle A2 centre (7.748685, 15.20765) radius 2
  circle A3 centre (9.295869, -14.314383) radius 2
  circle A4 centre (-17.044553, -0.893267) radius 2
  circle A5 centre (-7.748685, -15.20765) radius 2
  circle A6 centre (17.044553, 0.893267) radius 2
  circle A7 centre (-9.295869, 14.314383) radius 2
  point P0 (-1.315511, -25.101441)
extrude "Extrusion21" cut sketch "Sketch19" against normal blind 10
sketch "Sketch20" plane through (-1.315511, 25.101441, 20) normal (0, 0, -1) x (-1, 0, 0)
  circle A0 centre (0, 0) radius 24.135889
  circle A1 centre (-9.295869, 14.314383) radius 2
  circle A2 centre (17.044553, 0.893267) radius 2
  circle A3 centre (-7.748685, -15.20765) radius 2
  circle A4 centre (-17.044553, -0.893267) radius 2
  circle A5 centre (9.295869, -14.314383) radius 2
  circle A6 centre (7.748685, 15.20765) radius 2
  circle A7 centre (0, 0) radius 8
  circle A8 centre (0, 0) radius 24.95
  point P0 (-1.315511, -25.101441)
  dimension "d89" = 49.9
  constraints: 1 centre point, 1 coincident
  measures "d89" diameter of A8
extrude "Extrusion22" add sketch "Sketch20" against normal up to surface (7 mm away) contours A8
sketch "Sketch21" plane through (-1.315511, 25.101441, 42) normal (0, 0, 1) x (1, 0, 0)
  circle A0 centre (9.295869, 14.314383) radius 2
  circle A1 centre (17.044553, -0.893267) radius 2
  circle A2 centre (7.748685, -15.20765) radius 2
  circle A3 centre (-9.295869, -14.314383) radius 2
  circle A4 centre (-17.044553, 0.893267) radius 2
  circle A5 centre (-7.748685, 15.20765) radius 2
  circle A6 centre (0, 0) radius 70
  circle A7 centre (0, 0) radius 8
  line L0 (-7.506083, -11.214383) -> (-5.716297, -14.314383)
  line L1 (-5.716297, -14.314383) -> (-7.506083, -17.414383)
  line L2 (-7.506083, -17.414383) -> (-11.085655, -17.414383)
  line L3 (-11.085655, -17.414383) -> (-12.87544, -14.314383)
  line L4 (-12.87544, -14.314383) -> (-11.085655, -11.214383)
  line L5 (-11.085655, -11.214383) -> (-7.506083, -11.214383)
  line L6 (18.834339, -3.993267) -> (15.254768, -3.993267)
  line L7 (15.254768, -3.993267) -> (13.464982, -0.893267)
  line L8 (13.464982, -0.893267) -> (15.254768, 2.206733)
  line L9 (15.254768, 2.206733) -> (18.834339, 2.206733)
  line L10 (18.834339, 2.206733) -> (20.624125, -0.893267)
  line L11 (20.624125, -0.893267) -> (18.834339, -3.993267)
  line L12 (12.87544, 14.314383) -> (11.085655, 11.214383)
  line L13 (11.085655, 11.214383) -> (7.506083, 11.214383)
  line L14 (7.506083, 11.214383) -> (5.716297, 14.314383)
  line L15 (5.716297, 14.314383) -> (7.506083, 17.414383)
  line L16 (7.506083, 17.414383) -> (11.085655, 17.414383)
  line L17 (11.085655, 17.414383) -> (12.87544, 14.314383)
  line L18 (-18.834339, 3.993267) -> (-15.254768, 3.993267)
  line L19 (-15.254768, 3.993267) -> (-13.464982, 0.893267)
  line L20 (-13.464982, 0.893267) -> (-15.254768, -2.206733)
  line L21 (-15.254768, -2.206733) -> (-18.834339, -2.206733)
  line L22 (-18.834339, -2.206733) -> (-20.624125, 0.893267)
  line L23 (-20.624125, 0.893267) -> (-18.834339, 3.993267)
  line L24 (5.958899, -18.30765) -> (4.169113, -15.20765)
  line L25 (4.169113, -15.20765) -> (5.958899, -12.10765)
  line L26 (5.958899, -12.10765) -> (9.53847, -12.10765)
  line L27 (9.53847, -12.10765) -> (11.328256, -15.20765)
  line L28 (11.328256, -15.20765) -> (9.53847, -18.30765)
  line L29 (9.53847, -18.30765) -> (5.958899, -18.30765)
  line L30 (-5.958899, 18.30765) -> (-4.169113, 15.20765)
  line L31 (-4.169113, 15.20765) -> (-5.958899, 12.10765)
  line L32 (-5.958899, 12.10765) -> (-9.53847, 12.10765)
  line L33 (-9.53847, 12.10765) -> (-11.328256, 15.20765)
  line L34 (-11.328256, 15.20765) -> (-9.53847, 18.30765)
  line L35 (-9.53847, 18.30765) -> (-5.958899, 18.30765)
  circle A8 centre (3.242816, 61.876608) radius 4
  circle A9 centre (28.129943, -55.208122) radius 4
  circle A10 centre (-3.242816, -61.876608) radius 4
  circle A11 centre (-33.746665, -51.965307) radius 4
  circle A12 centre (33.746665, 51.965307) radius 4
  circle A13 centre (-28.129943, 55.208122) radius 4
  line L36 (-7.748685, 15.20765) -> (-5.064006, 13.65765)
  line L37 (-4.169113, 15.20765) -> (-5.958899, 12.10765)
  line L38 (-7.748685, 15.20765) -> (-4.717596, 13.45765)
  line L39 (-7.748685, 15.20765) -> (-10.433363, 16.75765)
  line L40 (-11.328256, 15.20765) -> (-9.53847, 18.30765)
  line L41 (-5.727959, 11.70765) -> (-9.769411, 11.70765)
  line L42 (-9.769411, 11.70765) -> (-11.790137, 15.20765)
  line L43 (-11.790137, 15.20765) -> (-9.769411, 18.70765)
  line L44 (-9.769411, 18.70765) -> (-5.727959, 18.70765)
  line L45 (-5.727959, 18.70765) -> (-3.707233, 15.20765)
  line L46 (-3.707233, 15.20765) -> (-5.727959, 11.70765)
  line L47 (-13.003102, 0.893267) -> (-15.023828, -2.606733)
  line L48 (-15.023828, 4.393267) -> (-13.003102, 0.893267)
  line L49 (-19.065279, 4.393267) -> (-15.023828, 4.393267)
  line L50 (-21.086005, 0.893267) -> (-19.065279, 4.393267)
  line L51 (-19.065279, -2.606733) -> (-21.086005, 0.893267)
  line L52 (-15.023828, -2.606733) -> (-19.065279, -2.606733)
  line L53 (-7.275143, -10.814383) -> (-5.254417, -14.314383)
  line L54 (-11.316595, -10.814383) -> (-7.275143, -10.814383)
  line L55 (-13.337321, -14.314383) -> (-11.316595, -10.814383)
  line L56 (-11.316595, -17.814383) -> (-13.337321, -14.314383)
  line L57 (-7.275143, -17.814383) -> (-11.316595, -17.814383)
  line L58 (-5.254417, -14.314383) -> (-7.275143, -17.814383)
  line L59 (5.727959, -11.70765) -> (9.769411, -11.70765)
  line L60 (3.707233, -15.20765) -> (5.727959, -11.70765)
  line L61 (5.727959, -18.70765) -> (3.707233, -15.20765)
  line L62 (9.769411, -18.70765) -> (5.727959, -18.70765)
  line L63 (11.790137, -15.20765) -> (9.769411, -18.70765)
  line L64 (9.769411, -11.70765) -> (11.790137, -15.20765)
  line L65 (13.003102, -0.893267) -> (15.023828, 2.606733)
  line L66 (15.023828, -4.393267) -> (13.003102, -0.893267)
  line L67 (19.065279, -4.393267) -> (15.023828, -4.393267)
  line L68 (21.086005, -0.893267) -> (19.065279, -4.393267)
  line L69 (19.065279, 2.606733) -> (21.086005, -0.893267)
  line L70 (15.023828, 2.606733) -> (19.065279, 2.606733)
  line L71 (7.275143, 10.814383) -> (5.254417, 14.314383)
  line L72 (11.316595, 10.814383) -> (7.275143, 10.814383)
  line L73 (13.337321, 14.314383) -> (11.316595, 10.814383)
  line L74 (11.316595, 17.814383) -> (13.337321, 14.314383)
  line L75 (7.275143, 17.814383) -> (11.316595, 17.814383)
  line L76 (5.254417, 14.314383) -> (7.275143, 17.814383)
  point P0 (1.315511, -25.101441)
  point P1 (-14.013465, 2.643267)
  point P2 (-9.295869, -10.814383)
  point P3 (4.717596, -13.45765)
  point P4 (14.013465, -2.643267)
  point P5 (9.295869, 10.814383)
  dimension "d92" = 3.5
  dimension "d95" = 360
  constraints: 78 end point, 3 midpoint, 1 coincident, 1 point on line, 92 other
  measures "d92" distance of L36.start L38.end
extrude "Extrusion23" cut sketch "Sketch21" against normal up to surface (10.4 mm away) contours A0 | A1 | A2 | A3 | A4 | A5 L36 L39 | A5 L39 L34 L35 L30 L31 L36 | L39 L36 A5 | A5 L36 L31 L32 L33 L34 L39 | L0 L1 L2 L3 L4 L5 | L6 L7 L8 L9 L10 L11 | L12 L13 L14 L15 L16 L17 | L18 L19 L20 L21 L22 L23 | L24 L25 L26 L27 L28 L29 | L41 L42 L43 L44 L45 L46 | L47 L52 L51 L50 L49 L48 | L53 L58 L57 L56 L55 L54 | L59 L64 L63 L62 L61 L60 | L65 L70 L69 L68 L67 L66 | L71 L76 L75 L74 L73 L72
sketch "Sketch22" plane through (-1.315511, 25.101441, 42) normal (0, 0, 1) x (1, 0, 0)
  line L0 (5.727959, -11.70765) -> (9.769411, -11.70765)
  line L1 (9.769411, -11.70765) -> (11.790137, -15.20765)
  line L2 (11.790137, -15.20765) -> (9.769411, -18.70765)
  line L3 (9.769411, -18.70765) -> (5.727959, -18.70765)
  line L4 (5.727959, -18.70765) -> (3.707233, -15.20765)
  line L5 (3.707233, -15.20765) -> (5.727959, -11.70765)
  line L6 (5.254417, 14.314383) -> (7.275143, 17.814383)
  line L7 (7.275143, 17.814383) -> (11.316595, 17.814383)
  line L8 (11.316595, 17.814383) -> (13.337321, 14.314383)
  line L9 (13.337321, 14.314383) -> (11.316595, 10.814383)
  line L10 (11.316595, 10.814383) -> (7.275143, 10.814383)
  line L11 (7.275143, 10.814383) -> (5.254417, 14.314383)
  line L12 (-13.003102, 0.893267) -> (-15.023828, -2.606733)
  line L13 (-15.023828, -2.606733) -> (-19.065279, -2.606733)
  line L14 (-19.065279, -2.606733) -> (-21.086005, 0.893267)
  line L15 (-21.086005, 0.893267) -> (-19.065279, 4.393267)
  line L16 (-19.065279, 4.393267) -> (-15.023828, 4.393267)
  line L17 (-15.023828, 4.393267) -> (-13.003102, 0.893267)
  line L18 (-5.254417, -14.314383) -> (-7.275143, -17.814383)
  line L19 (-7.275143, -17.814383) -> (-11.316595, -17.814383)
  line L20 (-11.316595, -17.814383) -> (-13.337321, -14.314383)
  line L21 (-13.337321, -14.314383) -> (-11.316595, -10.814383)
  line L22 (-11.316595, -10.814383) -> (-7.275143, -10.814383)
  line L23 (-7.275143, -10.814383) -> (-5.254417, -14.314383)
  line L24 (13.003102, -0.893267) -> (15.023828, 2.606733)
  line L25 (15.023828, 2.606733) -> (19.065279, 2.606733)
  line L26 (19.065279, 2.606733) -> (21.086005, -0.893267)
  line L27 (21.086005, -0.893267) -> (19.065279, -4.393267)
  line L28 (19.065279, -4.393267) -> (15.023828, -4.393267)
  line L29 (15.023828, -4.393267) -> (13.003102, -0.893267)
  line L30 (-9.769411, 11.70765) -> (-11.790137, 15.20765)
  line L31 (-11.790137, 15.20765) -> (-9.769411, 18.70765)
  line L32 (-9.769411, 18.70765) -> (-5.727959, 18.70765)
  line L33 (-5.727959, 18.70765) -> (-3.707233, 15.20765)
  line L34 (-3.707233, 15.20765) -> (-5.727959, 11.70765)
  line L35 (-5.727959, 11.70765) -> (-9.769411, 11.70765)
  circle A0 centre (0, 0) radius 70
  circle A1 centre (0, 0) radius 8
  circle A2 centre (3.242816, 61.876608) radius 4
  circle A3 centre (28.129943, -55.208122) radius 4
  circle A4 centre (-3.242816, -61.876608) radius 4
  circle A5 centre (-33.746665, -51.965307) radius 4
  circle A6 centre (33.746665, 51.965307) radius 4
  circle A7 centre (-28.129943, 55.208122) radius 4
  circle A8 centre (-7.748685, 15.20765) radius 2
  circle A9 centre (-7.748685, 15.20765) radius 4.1
  circle A10 centre (-17.044553, 0.893267) radius 4.1
  circle A11 centre (-9.295869, -14.314383) radius 4.1
  circle A12 centre (7.748685, -15.20765) radius 4.1
  circle A13 centre (17.044553, -0.893267) radius 4.1
  circle A14 centre (9.295869, 14.314383) radius 4.1
  point P0 (1.315511, -25.101441)
  dimension "d99" = 8.2
  dimension "d102" = 360
  constraints: 6 centre point, 1 coincident, 13 other
  measures "d99" diameter of A9
extrude "Extrusion24" cut sketch "Sketch22" against normal blind 5.4 contours L0 L1 L2 L3 L4 L5 | L6 L7 L8 L9 L10 L11 | L12 L13 L14 L15 L16 L17 | L18 L19 L20 L21 L22 L23 | L24 L25 L26 L27 L28 L29 | L30 L31 L32 L33 L34 L35 | A8 | A9 | A10 | A11 | A12 | A13 | A14
sketch "Szkic24" plane through (-1.315511, 25.101441, 42) normal (0, 0, 1) x (1, 0, 0)
  circle A0 centre (9.295869, 14.314383) radius 4.1
  circle A1 centre (9.295869, 14.314383) radius 2
  circle A2 centre (9.295869, 14.314383) radius 5
  point P0 (1.315511, -25.101441)
  dimension "d118" = 10
  constraints: 1 centre point, 1 coincident
  measures "d118" diameter of A2
extrude "Wyciągnięcie proste26" cut sketch "Szkic24" against normal up to surface (5.4 mm away) contours A0 | A1 | A2
pattern_circular "Szyk kołowy1" count 6 over 360 about axis through (-1.315511, 25.101441, 0) along (0, 0, 1) of "Wyciągnięcie proste26"
sketch "Szkic25" plane through (-1.315511, 25.101441, 42) normal (0, 0, 1) x (1, 0, 0)
  circle A0 centre (17.044553, -0.893267) radius 5
  circle A1 centre (7.748685, -15.20765) radius 5
  circle A2 centre (-9.295869, -14.314383) radius 5
  circle A3 centre (-17.044553, 0.893267) radius 5
  circle A4 centre (-7.748685, 15.20765) radius 5
  circle A5 centre (9.295869, 14.314383) radius 5
  circle A6 centre (0, 0) radius 70
  circle A7 centre (0, 0) radius 8
  circle A8 centre (3.242816, 61.876608) radius 4
  circle A9 centre (28.129943, -55.208122) radius 4
  circle A10 centre (-3.242816, -61.876608) radius 4
  circle A11 centre (-33.746665, -51.965307) radius 4
  circle A12 centre (33.746665, 51.965307) radius 4
  circle A13 centre (-28.129943, 55.208122) radius 4
  circle A14 centre (33.746665, 51.965307) radius 4.25
  circle A15 centre (3.242816, 61.876608) radius 4.25
  circle A16 centre (-28.129943, 55.208122) radius 4.25
  circle A17 centre (-33.746665, -51.965307) radius 4
  circle A18 centre (-33.746665, -51.965307) radius 4.25
  circle A19 centre (-3.242816, -61.876608) radius 4.25
  circle A20 centre (28.129943, -55.208122) radius 4.25
  point P0 (1.315511, -25.101441)
  dimension "d124" = 8.5
  dimension "d125" = 8.5
  dimension "d126" = 8.5
  dimension "d127" = 8.5
  dimension "d128" = 8.5
  dimension "d129" = 8.5
  constraints: 6 centre point, 6 coincident
  measures "d124" diameter of A14
  measures "d125" diameter of A15
  measures "d126" diameter of A16
  measures "d127" diameter of A18
  measures "d128" diameter of A19
  measures "d129" diameter of A20
extrude "Wyciągnięcie proste27" cut sketch "Szkic25" against normal through all contours A8 | A9 | A10 | A11 | A12 | A13 | A14 | A15 | A16 | A18 | A19 | A20
chamfer "Faza2" distance 1.5 angle 45 30 edges at (-35.637, 80.634, 27) (-26.0687, 85.5093, 27) (-23.254, 79.9851, 27) (-26.6307, 74.7853, 27) (-32.8222, 75.1098, 27) (-3.5969, 84.1633, 27) (-3.2725, 90.3548, 27) (1.6028, 80.7865, 27) (7.1271, 83.6013, 27) (7.4515, 89.7928, 27) (26.2397, 77.3912, 27) (29.0544, 71.867, 27) (35.2459, 71.5425, 27) (29.6164, 82.591, 27) (38.6227, 76.7423, 27) (33.0059, -30.4312, 27) (23.4377, -35.3064, 27) (20.6229, -29.7822, 27) (23.9997, -24.5824, 27) (30.1912, -24.9069, 27) (0.9659, -33.9604, 27) (0.6414, -40.1519, 27) (-9.7581, -33.3984, 27) (-10.0826, -39.5899, 27) (-4.2338, -30.5837, 27) (-41.2537, -26.5394, 27) (-37.8769, -21.3396, 27) (-31.6854, -21.6641, 27) (-28.8707, -27.1883, 27) (-32.2474, -32.3881, 27)
fillet "Zaokrąglenie5" radius 2 6 edges at (2.9804, 39.4158, 42) (13.229, 28.5383, 42) (8.9332, 14.2239, 42) (-5.6114, 10.7871, 42) (-15.8601, 21.6646, 42) (-11.5642, 35.979, 42)
chamfer "Faza3" distance 1 angle 45 6 edges at (28.1812, 77.0667, 42) (-2.3227, 86.978, 42) (-33.6955, 80.3096, 42) (22.5644, -30.1067, 42) (-8.8083, -36.7752, 42) (-39.3122, -26.8639, 42)